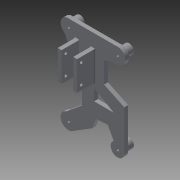
# Autodesk Inventor part: gimbal_controller_holder
Saved by Autodesk Inventor 2015 SP1 (Build 190203100, 203)
## iProperties
Created: 2015-08-17
Part Number: gimbal_controller_holder
Material: Generic
Document SubType Name: Modeling
Designer: Alexandre Cherpillod
Density: 1 g/cm^3
Appearance: Default
Author: Alexandre Cherpillod
Autodesk Inventor part; units mm, degrees
ref_plane "YZ Plane" through (0, 0, 0) normal (1, 0, 0) x (0, 1, 0)
ref_plane "XZ Plane" through (0, 0, 0) normal (0, 1, 0) x (-1, 0, 0)
ref_plane "XY Plane" through (0, 0, 0) normal (0, 0, 1) x (1, 0, 0)
sketch "Sketch1" plane through (0, 0, 0) normal (0, 1, 0) x (-1, 0, 0)
  line L0 (0, 0) -> (25.3, 0) construction
  line L1 (25.3, 0) -> (25.3, -42) construction
  line L2 (25.3, -42) -> (0, -42) construction
  line L3 (0, -42) -> (0, 0) construction
  circle A0 centre (25.3, 0) radius 2.5
  circle A1 centre (0, 0) radius 2.5
  circle A2 centre (0, -42) radius 2.5
  circle A3 centre (25.3, -42) radius 2.5
  dimension "d0" = 25.3
  dimension "d1" = 42
  dimension "d2" = 5
  dimension "d3" = 5
  dimension "d4" = 5
  dimension "d5" = 5
  constraints: 8 end point, 4 centre point, 4 coincident, 2 parallel, 1 horizontal, 1 perpendicular
  measures "d0" distance of L1.end L2.end
  measures "d1" distance of L0.end L1.end
  measures "d2" diameter of A0
  measures "d3" diameter of A1
  measures "d4" diameter of A2
  measures "d5" diameter of A3
extrude "Extrusion1" add sketch "Sketch1" along normal blind 6
sketch "Sketch2" plane through (0, 0, 0) normal (0, 1, 0) x (-1, 0, 0)
  circle A0 centre (0, 0) radius 2.5 projected
  arc A1 (0.8438, 3.91) -> (-0.7933, -3.9205) centre (0, 0) ccw
  arc A2 (27.3626, -3.4272) -> (24.4562, 3.91) centre (25.3, 0) ccw
  circle A3 centre (25.3, -42) radius 2.5 projected
  arc A4 (22.5627, -44.9167) -> (26.3151, -38.1309) centre (25.3, -42) ccw
  circle A5 centre (0, -42) radius 2.5 projected
  arc A6 (-3.5, -42) -> (1.9296, -39.08) centre (0, -42) ccw
  line L0 (26.3151, -38.1309) -> (18.3, -31.5476)
  line L1 (0.8438, 3.91) -> (24.4562, 3.91)
  line L2 (6.9132, -16.448) -> (6.9132, -5.4484)
  line L3 (6.9132, -5.4484) -> (-0.7933, -3.9205)
  line L4 (18.3, -31.5476) -> (18.3, -18.0196)
  line L5 (-3.5, -42) -> (-3.5, -21.4061)
  line L6 (-3.5, -21.4061) -> (6.9132, -16.448)
  line L7 (22.5627, -44.9167) -> (13.1542, -39.1017)
  line L8 (13.1542, -39.1017) -> (11.1047, -33.8253)
  line L9 (11.1047, -33.8253) -> (5.0372, -33.4161)
  line L10 (35.6, -30.5) -> (19.8, -30.5) construction
  line L11 (19.8, -30.5) -> (19.8, -14.4) construction
  line L12 (19.8, -14.4) -> (35.6, -14.4) construction
  line L13 (35.6, -14.4) -> (35.6, -30.5) construction
  circle A7 centre (8, -39.2) radius 4.55 construction
  line L14 (-2.3049, -15.9586) -> (4, -15.9586) construction
  line L15 (4, -15.9586) -> (4, -6.2) construction
  line L16 (4, -6.2) -> (-2.3049, -6.2) construction
  line L17 (-2.3049, -6.2) -> (-2.3049, -15.9586) construction
  line L18 (5.0372, -33.4161) -> (1.9296, -39.08)
  line L19 (12.0305, -26.4894) -> (1.9134, -26.4894)
  line L20 (1.9134, -26.4894) -> (12.0305, -20.5783)
  line L21 (12.0305, -20.5783) -> (12.0305, -26.4894)
  line L22 (18.3, -18.0196) -> (20.2183, -18.0196)
  line L23 (20.2183, -18.0196) -> (27.3626, -3.4272)
  dimension "d8" = 8
  dimension "d9" = 8
  dimension "d10" = 8
  dimension "d11" = 7
  dimension "d15" = 7
  dimension "d18" = 15.8
  dimension "d19" = 11.5
  dimension "d20" = 16.1
  dimension "d21" = 2.8
  dimension "d22" = 8
  dimension "d23" = 9.1
  dimension "d24" = 6.2
  dimension "d25" = 4
  dimension "d26" = 9.7586
  dimension "d27" = 6.3049
  dimension "d28" = 5.5
  constraints: 48 end point, 8 point on circle, 5 centre point, 4 perpendicular, 3 coincident, 3 horizontal, 3 parallel, 2 vertical, 1 horizontal alignment, 1 tangent, 1 vertical alignment
  measures "d8" diameter of A1
  measures "d9" diameter of A2
  measures "d10" diameter of A4
  measures "d11" diameter of A6
  measures "d15" horizontal distance of L0.end A4.centre
  measures "d18" distance between parallel lines of L13 L11
  measures "d19" distance from line of A4.centre L10
  measures "d20" distance between parallel lines of L12 L10
  measures "d21" vertical distance of A7.centre A6.centre
  measures "d22" horizontal distance of A7.centre A6.centre
  measures "d23" diameter of A7
  measures "d24" distance from line of point (0, 0) L16
  measures "d25" distance from line of point (0, 0) L15
  measures "d26" distance between parallel lines of L14 L16
  measures "d27" distance between parallel lines of L17 L15
  measures "d28" distance from line of L11 A3.centre
extrude "Extrusion2" add sketch "Sketch2" along normal blind 2
hole "Hole1" at (-25.3, 6, 0) direction (0, -1, 0) diameter 1.4 depth 8 tip angle 118
hole "Hole2" at (-25.3, 6, -42) direction (0, -1, 0) diameter 1.4 depth 8 tip angle 118
hole "Hole3" at (0, 6, -42) direction (0, -1, 0) diameter 1.4 depth 8 tip angle 118
hole "Hole4" at (0, 6, 0) direction (0, -1, 0) diameter 1.4 depth 8 tip angle 118
sketch "Sketch3" plane through (0, 0, 0) normal (0, 1, 0) x (-1, 0, 0)
  line L0 (21.8, -18.05) -> (19.8, -18.05)
  line L1 (19.8, -18.05) -> (19.8, -3.05)
  line L2 (19.8, -3.05) -> (21.8, -3.05)
  line L3 (21.8, -3.05) -> (21.8, -18.05)
  circle A0 centre (25.3, 0) radius 0.7 construction
  circle A1 centre (25.3, -42) radius 0.7 construction
  circle A2 centre (0, -42) radius 0.7 construction
  circle A3 centre (0, 0) radius 0.7 construction
  line L4 (13.8, -18.05) -> (11.8, -18.05)
  line L5 (11.8, -18.05) -> (11.8, -3.05)
  line L6 (11.8, -3.05) -> (13.8, -3.05)
  line L7 (13.8, -3.05) -> (13.8, -18.05)
  dimension "d69" = 2
  dimension "d70" = 15
  dimension "d73" = 3.5
  dimension "d74" = 18.05
  dimension "d79" = 2
  dimension "d80" = 6
  constraints: 16 end point, 4 parallel, 2 horizontal, 2 perpendicular
  measures "d69" distance of L1.end L2.end
  measures "d70" distance of L2.end L0.start
  measures "d73" distance from line of A0.centre L3
  measures "d74" distance from line of A0.centre L0
  measures "d79" distance of L5.end L6.end
  measures "d80" distance between parallel lines of L7 L1
extrude "Extrusion3" add sketch "Sketch3" along normal blind 2 and the other way blind 9
fillet "Fillet1" radius 1 3 edges at (-22.8, 2, -42) (2.5, 2, 0) (-22.8, 2, 0)
sketch "Sketch4" plane through (-11.8, -9, -3.05) normal (1, 0, 0) x (0, 0, -1)
  circle A0 centre (12.5084, 2.25) radius 0.75
  circle A1 centre (2.5084, 2.25) radius 0.75
  line L0 (18.3561, 9) -> (13.398, 9) projected
  point P0 (-3.05, 9)
  dimension "d83" = 1.5
  dimension "d84" = 10
  dimension "d85" = 6.75
  constraints: 2 centre point, 1 equal radius, 1 horizontal alignment
  measures "d83" diameter of A1
  measures "d84" distance of A1.centre A0.centre
  measures "d85" distance from line of L0 A0.centre
extrude "Extrusion4" cut sketch "Sketch4" against normal through all
fillet "Fillet2" radius 0.5 5 edges at (-11.8, 0, -10.55) (-21.8, 0, -8.9195) (-20.8, 0, -3.05) (-12.8, 0, -3.05) (-12.8, 0, -18.05)
body "Solid1"
